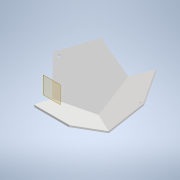
# Autodesk Inventor part: dodecahedron
Saved by Autodesk Inventor 2020.2 (Build 242310000, 310)
## iProperties
Created: 2020-01-17
Part Number: dodecahedron
Material: Generic
Document SubType Name: Modeling
Designer: Bardo91
Density: 1 g/cm^3
Appearance: Default
Author: Bardo91
Autodesk Inventor part; units mm, degrees
ref_plane "YZ Plane" through (0, 0, 0) normal (1, 0, 0) x (0, 1, 0)
ref_plane "XZ Plane" through (0, 0, 0) normal (0, 1, 0) x (-1, 0, 0)
ref_plane "Work Plane1" through (0, 0, 44.5407) normal (0, 0, 1) x (1, 0, 0)
sketch "Sketch2" plane through (0, 0, 44.5407) normal (0, 0, 1) x (1, 0, 0)
  line L0 (0, 34.026) -> (32.3607, 10.5146)
  line L1 (32.3607, 10.5146) -> (20, -27.5276)
  line L2 (20, -27.5276) -> (-20, -27.5276)
  line L3 (-20, -27.5276) -> (-32.3607, 10.5146)
  line L4 (-32.3607, 10.5146) -> (0, 34.026)
  point P0 (0, 0)
  point P1 (0, 0)
  dimension "d2" = 40
  constraints: 10 end point, 1 coincident, 11 other
  measures "d2" distance of L1.end L2.end
loft "Loft1" add profiles "Sketch2" section 2 point at (0, 0, 0)
mirror "Mirror1" about plane through (32.3607, 10.5146, 44.5407) normal (0.809017, -0.2628656, -0.5257311) of "Loft1"
mirror "Mirror2" about plane through (20, -27.5276, 44.5407) normal (0, -0.8506508, -0.5257311) of "Loft1"
mirror "Mirror3" about plane through (-20, -27.5276, 44.5407) normal (-0.809017, -0.2628656, -0.5257311) of "Loft1"
mirror "Mirror4" about plane through (-32.3607, 10.5146, 44.5407) normal (-0.5, 0.688191, -0.5257311) of "Loft1"
mirror "Mirror5" about plane through (0, 34.026, 44.5407) normal (0.5, 0.688191, -0.5257311) of "Loft1"
mirror "Mirror6" about plane through (-52.3607, -17.013, -10.5146) normal (0.309017, -0.4253254, -0.8506508) of "Loft1", "Mirror3"
mirror "Mirror7" about plane through (-52.3607, 17.013, 10.5146) normal (0, 0.5257311, -0.8506508) of "Loft1", "Mirror3"
mirror "Mirror8" about plane through (52.3607, -17.013, -10.5146) normal (0, 0.5257311, -0.8506508) of "Loft1", "Mirror1"
mirror "Mirror9" about plane through (20, 27.5276, -44.5407) normal (-0.809017, -0.2628656, -0.5257311) of "Loft1", "Mirror1", "Mirror8"
shell "Shell1" thickness 2 removed faces 9 at (-17.4536, 35.3648, 21.8566) at (0, 36.7035, -26.1889) at (21.5738, 29.6938, 26.1889) at (-6.6667, -2.1661, 44.5407) at (39.0273, -5.671, 21.8566) at (39.0273, 17.013, -14.8469) at (-4.1202, -5.671, -44.5407) at (-41.5738, 9.1759, -14.8469) at (-39.0273, -5.671, 21.8566)
sketch "Sketch3" plane through (-32.3607, -44.5407, 10.5146) normal (-0.5257311, -0.7236068, -0.4472136) x (0.809017, -0.2628656, -0.5257311)
  line L0 (-13.5363, -38.4242) -> (20, -62.7897) projected
  line L1 (-13.5363, -38.4242) -> (-8.0063, -42.442)
  line L2 (-1.4531, -1.2361) -> (-13.5363, -38.4242) projected
  line L3 (-13.5363, -38.4242) -> (-11.5295, -32.2482)
  line L4 (-13.5363, -38.4242) -> (-7.8299, -36.5701)
  circle A0 centre (-7.8299, -36.5701) radius 1.5
  point P0 (20, -27.5276)
  dimension "d8" = 6
  dimension "d9" = 54
  dimension "d10" = 108
  dimension "d11" = 3
  constraints: 6 end point, 2 point on line, 1 centre point, 1 coincident
  measures "d8" distance of L0.start L4.end
  measures "d9" angle of L4 L0
  measures "d10" angle of L2 L0
  measures "d11" diameter of A0
extrude "Extrusion1" cut sketch "Sketch3" against normal through all
sketch "Sketch4" plane through (0, -55.0553, -10.5146) normal (0.5257311, -0.7236068, -0.4472136) x (0.809017, 0.2628656, 0.5257311)
  line L0 (52.3607, -38.0423) -> (53.5363, -38.4242) projected
  line L1 (53.5363, -38.4242) -> (50.6191, -40.5437)
  line L2 (20, -62.7897) -> (53.5363, -38.4242) projected
  line L3 (53.5363, -38.4242) -> (53.5363, -38.4242)
  line L4 (53.5363, -38.4242) -> (41.4531, -1.2361) projected
  line L5 (53.5363, -38.4242) -> (47.8299, -36.5701)
  circle A0 centre (47.8299, -36.5701) radius 1.5
  point P0 (20, -27.5276)
  dimension "d14" = 6
  dimension "d15" = 108
  dimension "d16" = 54
  dimension "d17" = 3
  constraints: 6 end point, 2 point on line, 1 centre point, 1 coincident
  measures "d14" distance of L0.end L5.end
  measures "d15" angle of L1 L3
  measures "d16" angle of L4 L5
  measures "d17" diameter of A0
extrude "Extrusion2" cut sketch "Sketch4" against normal through all
equation "\"d9\" = 0.5 * d10"
body "Solid1"
